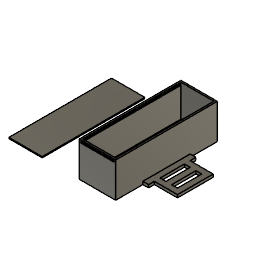
Ethan_TB_CaseV3 (Autodesk Fusion 360 design; units mm, degrees)
part number: 2026-03-08-13-35-21-563
Autodesk Fusion 360 part; units mm, degrees
sketch "Sketch1" plane through (0, 0, 0) normal (0, 0, 1) x (1, 0, 0)
  line L0 (-10, 20) -> (53.2, 20)
  line L1 (53.2, 20) -> (53.2, -156.2)
  line L2 (53.2, -156.2) -> (-10, -156.2)
  line L3 (-10, -156.2) -> (-10, 20)
  dimension "d1" = 63.2
  dimension "d2" = 176.2
  constraint horizontal L0
  constraint vertical L1
  constraint horizontal L2
  constraint vertical L3
  measures "d1" distance of L0.start L0.end
  measures "d2" distance of L0.start L2.end
extrude "Extrude1" add sketch "Sketch1" along normal blind 60.5 makes body 1
sketch "Sketch2" plane through (0, 0, 60.5) normal (0, 0, 1) x (-1, 0, 0)
  line L0 (10, 156.2) -> (-53.2, 156.2)
  line L1 (-53.2, 156.2) -> (-53.2, -20)
  line L2 (-53.2, -20) -> (10, -20)
  line L3 (10, -20) -> (10, 156.2)
  line L4 (7, -17) -> (-50.2, -17)
  line L5 (-50.2, -17) -> (-50.2, 153.2)
  line L6 (-50.2, 153.2) -> (7, 153.2)
  line L7 (7, 153.2) -> (7, -17)
  dimension "d10" = 57.2
  dimension "d11" = 170.2
  dimension "d12" = 3
  dimension "d13" = 3
  constraint horizontal L4
  constraint vertical L5
  constraint horizontal L6
  constraint vertical L7
  measures "d10" distance of L4.start L4.end
  measures "d11" distance of L4.end L5.end
  measures "d12" distance of L3 L7
  measures "d13" distance of L2 L4
extrude "Extrude3" cut sketch "Sketch2" against normal blind 55.5 contours L4 L5 L6 L7 bodies 1
sketch "Sketch4" plane through (0, -156.2, 0) normal (0, -1, 0) x (1, 0, 0)
  line L0 (-10, 0) -> (53.2, 0)
  line L1 (53.2, 0) -> (53.2, 60.5)
  line L2 (53.2, 60.5) -> (-10, 60.5)
  line L3 (-10, 60.5) -> (-10, 0)
  line L4 (-7.5, 58) -> (50.5, 58)
  line L5 (50.5, 58) -> (50.5, 56)
  line L6 (50.5, 56) -> (-7.5, 56)
  line L7 (-7.5, 56) -> (-7.5, 58)
  line L8 (50.2, 60.5) -> (-7, 60.5)
  line L9 (-131.921, 1.9) -> (-74.021, 1.9)
  line L10 (-74.021, 1.9) -> (-74.021, 0)
  line L11 (-74.021, 0) -> (-131.921, 0)
  line L12 (-131.921, 0) -> (-131.921, 1.9)
  dimension "d22" = 58
  dimension "d23" = 2
  dimension "d24" = 2.5
  dimension "d25" = 2.5
  dimension "d40" = 1.9
  dimension "d41" = 57.9
  constraint horizontal L4
  constraint vertical L5
  constraint horizontal L6
  constraint vertical L7
  constraint horizontal L9
  constraint vertical L10
  constraint horizontal L11
  constraint vertical L12
  constraint collinear L0 L11
  measures "d22" distance of L4.start L4.end
  measures "d23" distance of L4.start L6.end
  measures "d24" distance of L4 L8
  measures "d25" distance of L3 L7
  measures "d40" distance of L9 L11
  measures "d41" distance of L9.start L9.end
extrude "Extrude4" cut sketch "Sketch4" against normal blind 173.2 contours L4 L5 L6 L7 | L9 L10 L11 L12 bodies 1
extrude "Extrude6" add sketch "Sketch4" against normal blind 178 separate body contours L9 L10 L11 L12 makes body 2
sketch "Sketch5" plane through (0, 0, 0) normal (0, 0, -1) x (1, 0, 0)
  line L0 (53.2, 156.2) -> (-10, 156.2)
  line L1 (-10, 156.2) -> (-10, -20)
  line L2 (-10, -20) -> (53.2, -20)
  line L3 (-10, 37.1) -> (-60, 37.1)
  line L4 (-60, 37.1) -> (-60, 99.1)
  line L5 (-60, 99.1) -> (-10, 99.1)
  line L6 (-10, 99.1) -> (-10, 37.1)
  line L7 (53.2, -20) -> (-10, -20)
  line L8 (-50, 47.1) -> (-40, 47.1)
  line L9 (-40, 47.1) -> (-40, 89.1)
  line L10 (-40, 89.1) -> (-50, 89.1)
  line L11 (-50, 89.1) -> (-50, 47.1)
  line L12 (-30, 47.1) -> (-20, 47.1)
  line L13 (-20, 47.1) -> (-20, 89.1)
  line L14 (-20, 89.1) -> (-30, 89.1)
  line L15 (-30, 89.1) -> (-30, 47.1)
  line L16 (21.6, 39.3466) -> (21.6, 140)
  line L17 (-10, -20) -> (-10, 156.2)
  line L18 (83.2, 47.1) -> (83.2, 89.1)
  line L19 (73.2, 89.1) -> (73.2, 47.1)
  line L20 (73.2, 47.1) -> (63.2, 47.1)
  line L21 (53.2, 37.1) -> (103.2, 37.1)
  line L22 (83.2, 89.1) -> (93.2, 89.1)
  line L23 (63.2, 47.1) -> (63.2, 89.1)
  line L24 (53.2, 99.1) -> (53.2, 37.1)
  line L25 (63.2, 89.1) -> (73.2, 89.1)
  line L26 (103.2, 37.1) -> (103.2, 99.1)
  line L27 (93.2, 89.1) -> (93.2, 47.1)
  line L28 (103.2, 99.1) -> (53.2, 99.1)
  line L29 (93.2, 47.1) -> (83.2, 47.1)
  line L30 (-10, 37.1) -> (-20, 37.1)
  line L31 (-20, 37.1) -> (-20, 27.1)
  line L32 (-20, 27.1) -> (-10, 27.1)
  line L33 (-10, 27.1) -> (-10, 37.1)
  line L34 (-10, 99.1) -> (-20, 99.1)
  line L35 (-20, 99.1) -> (-20, 109.1)
  line L36 (-20, 109.1) -> (-10, 109.1)
  line L37 (-10, 109.1) -> (-10, 99.1)
  line L38 (83.2, 89.1) -> (93.2, 89.1)
  line L39 (63.2, 109.1) -> (53.2, 109.1)
  line L40 (53.2, 99.1) -> (63.2, 99.1)
  line L41 (83.2, 47.1) -> (83.2, 89.1)
  line L42 (53.2, 37.1) -> (103.2, 37.1)
  line L43 (63.2, 27.1) -> (53.2, 27.1)
  line L44 (93.2, 47.1) -> (83.2, 47.1)
  line L45 (73.2, 89.1) -> (73.2, 47.1)
  line L46 (63.2, 99.1) -> (63.2, 109.1)
  line L47 (53.2, 37.1) -> (63.2, 37.1)
  line L48 (73.2, 47.1) -> (63.2, 47.1)
  line L49 (103.2, 99.1) -> (53.2, 99.1)
  line L50 (53.2, 99.1) -> (53.2, 37.1)
  line L51 (53.2, 27.1) -> (53.2, 37.1)
  line L52 (63.2, 89.1) -> (73.2, 89.1)
  line L53 (63.2, 47.1) -> (63.2, 89.1)
  line L54 (93.2, 89.1) -> (93.2, 47.1)
  line L55 (53.2, 109.1) -> (53.2, 99.1)
  line L56 (63.2, 37.1) -> (63.2, 27.1)
  dimension "d28" = 57.1
  dimension "d29" = 62
  dimension "d30" = 50
  dimension "d31" = 42
  dimension "d32" = 10
  dimension "d34" = 10
  dimension "d35" = 10
  dimension "d36" = 10
  dimension "d37" = 31.6
  dimension "d44" = 10
  dimension "d45" = 10
  dimension "d46" = 10
  dimension "d47" = 10
  constraint horizontal L3
  constraint vertical L4
  constraint horizontal L5
  constraint vertical L6
  constraint coincident L1 L3.start
  constraint horizontal L8
  constraint vertical L9
  constraint horizontal L10
  constraint vertical L11
  constraint horizontal L12
  constraint vertical L13
  constraint horizontal L14
  constraint vertical L15
  constraint equal L8 L12
  constraint equal L11 L15
  constraint collinear L8 L12
  constraint perpendicular L7 L16
  constraint symmetric L3.start L16 L21.start
  constraint symmetric L3.end L16 L21.end
  constraint symmetric L4.end L16 L26.end
  constraint symmetric L5.end L16 L24.start
  constraint symmetric L8.start L16 L27.end
  constraint symmetric L8.end L16 L18.start
  constraint symmetric L9.end L16 L18.end
  constraint symmetric L10.end L16 L22.end
  constraint symmetric L12.start L16 L19.end
  constraint symmetric L12.end L16 L20.end
  constraint symmetric L13.end L16 L23.end
  constraint symmetric L14.end L16 L19.start
  constraint horizontal L30
  constraint vertical L31
  constraint horizontal L32
  constraint vertical L33
  constraint horizontal L34
  constraint vertical L35
  constraint horizontal L36
  constraint vertical L37
  constraint symmetric L16 L30.end L47.end
  constraint symmetric L16 L31.end L43.start
  constraint symmetric L16 L32.end L43.end
  constraint symmetric L16 L34.end L40.end
  constraint symmetric L16 L35.end L39.start
  constraint symmetric L16 L36.end L39.end
  measures "d28" distance of L3 L7
  measures "d29" distance of L3.end L4.end
  measures "d30" distance of L3.start L3.end
  measures "d31" distance of L8.start L10.end
  measures "d32" distance of L8.start L8.end
  measures "d34" distance of L9 L15
  measures "d35" distance of L4 L11
  measures "d36" distance of L3 L8
  measures "d37" distance of L16 L17
  measures "d44" distance of L3.start L30.end
  measures "d45" distance of L3.start L32.end
  measures "d46" distance of L5.end L34.end
  measures "d47" distance of L5.end L36.end
extrude "Extrude5" add sketch "Sketch5" against normal blind 5 bodies 1
sketch "Sketch6" plane through (0, -156.2, 0) normal (0, -1, 0) x (1, 0, 0)
  line L0 (50.5, 56) -> (-7.5, 56)
  line L1 (-7.5, 56) -> (-7.5, 58)
  line L2 (-7.5, 58) -> (50.5, 58)
  line L3 (-10, 0) -> (53.2, 0)
  line L4 (53.2, 0) -> (53.2, 60.5)
  line L5 (53.2, 60.5) -> (-10, 60.5)
  line L6 (-10, 60.5) -> (-10, 0)
  line L7 (50.5, 58) -> (50.5, 56)
equation "d2 = 18.02 cm - 0.4 cm"
equation "d8 = 6.45 cm - 0.4 cm"
equation "d22 = 6.2 cm - 0.4 cm"
equation "d40 = 2 mm - 0.1 mm"
equation "d41 = 62 mm - 0.1 mm - 0.4 cm"
